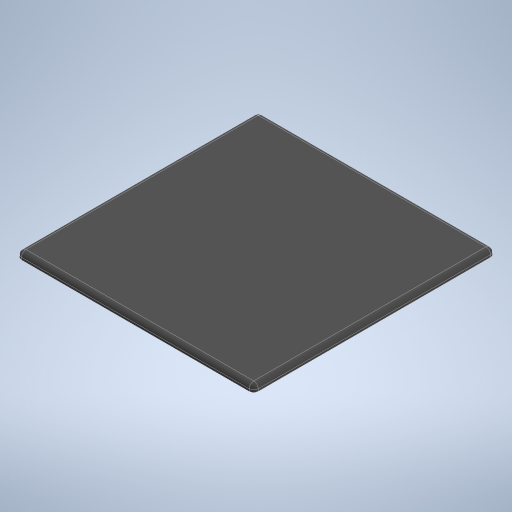
# Autodesk Inventor part: Lid
Saved by Autodesk Inventor 2023 (Build 270158000, 158)
## iProperties
Created: 2023-03-26
Part Number: Lid
Material: Generic
Document SubType Name: Modeling
Designer: Ahmed Nazir
Density: 1 g/cm^3
Appearance: Default
Author: Ahmed Nazir
Autodesk Inventor part; units mm, degrees
ref_plane "YZ Plane" through (0, 0, 0) normal (1, 0, 0) x (0, 1, 0)
ref_plane "XZ Plane" through (0, 0, 0) normal (0, 1, 0) x (-1, 0, 0)
ref_plane "XY Plane" through (0, 0, 0) normal (0, 0, 1) x (1, 0, 0)
sketch "Sketch1" plane through (0, 0, 0) normal (0, 1, 0) x (-1, 0, 0)
  line L0 (49, 50) -> (-49, 50)
  line L1 (-49, 50) -> (-49, -50)
  line L2 (-49, -50) -> (49, -50)
  line L3 (49, -50) -> (49, 50)
  line L4 (49, 50) -> (-49, -50) construction
  line L5 (-49, 50) -> (49, -50) construction
  line L6 (52, -53) -> (-52, -53)
  line L7 (-52, -53) -> (-52, 53)
  line L8 (-52, 53) -> (52, 53)
  line L9 (52, 53) -> (52, -53)
  line L10 (46, 47) -> (-46, 47)
  line L11 (-46, 47) -> (-46, -47)
  line L12 (-46, -47) -> (46, -47)
  line L13 (46, -47) -> (46, 47)
  point P0 (0, 0)
  dimension "d0" = 98
  dimension "d1" = 100
  dimension "d2" = 3
  dimension "d3" = 3
  constraints: 28 end point, 6 parallel, 3 perpendicular, 2 midpoint, 1 horizontal, 6 other
  measures "d0" distance of L2.end L1.end
  measures "d1" distance of L1.end L0.end
  measures "d2" distance between parallel lines of L2 L6
  measures "d3" distance between parallel lines of L3 L13
extrude "Extrusion1" add sketch "Sketch1" along normal blind 3 contours L3 L2 L1 L0 | L6 L7 L8 L9 | L13 L12 L11 L10
extrude "Extrusion2" add sketch "Sketch1" against normal blind 3 contours L3 L2 L1 L0
sketch "Sketch2" plane through (0, -3, 0) normal (0, -1, 0) x (1, 0, 0)
  line L0 (-49, -50) -> (49, -50) projected
  circle A0 centre (49, -50) radius 2.5
  circle A1 centre (-49, -50) radius 2.5
  line L1 (49, 50) -> (49, -50) projected
  circle A2 centre (49, 50) radius 2.5
  line L2 (49, 50) -> (-49, 50) projected
  circle A3 centre (-49, 50) radius 2.5
  point P0 (0, 0)
  dimension "d8" = 5
  dimension "d9" = 5
  dimension "d10" = 5
  dimension "d12" = 5
  constraints: 4 centre point, 1 coincident
  measures "d8" diameter of A0
  measures "d9" diameter of A1
  measures "d10" diameter of A2
  measures "d12" diameter of A3
extrude "Extrusion3" cut sketch "Sketch2" against normal blind 4.5
fillet "Fillet1" radius 2 8 edges at (-52, 1.5, 53) (0, 3, 53) (-52, 3, 0) (52, 1.5, 53) (52, 3, 0) (52, 1.5, -53) (0, 3, -53) (-52, 1.5, -53)
body "Solid1"
